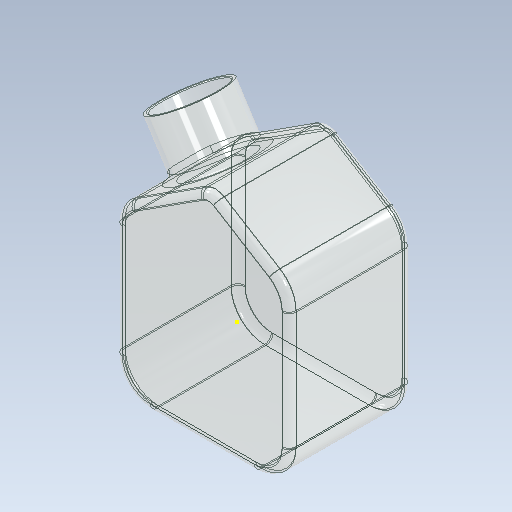
# Autodesk Inventor part: MediumBottle
Saved by Autodesk Inventor 2020 (Build 240168000, 168)
## iProperties
Created: 2023-04-07
Part Number: MediumBottle
Material: Glass
Document SubType Name: Modeling
Designer: DSOB
Density: 2.18 g/cm^3
Appearance: Clear
Author: DSOB
Autodesk Inventor part; units mm, degrees
ref_plane "XZ Plane" through (0, 0, 0) normal (0, 1, 0) x (-1, 0, 0)
ref_plane "XY Plane" through (0, 0, 0) normal (0, 0, 1) x (1, 0, 0)
sketch "Sketch1" plane through (0, 0, 0) normal (0, 0, 1) x (1, 0, 0)
  line L0 (0, 20) -> (0, 84.7083)
  line L1 (7.8208, 99.0171) -> (47.7041, 124.6026)
  line L2 (58.3547, 124.696) -> (90.5021, 104.8604)
  line L3 (100, 87.8397) -> (100, 20)
  line L4 (80, 0) -> (20, 0)
  arc A0 (0, 20) -> (20, 0) centre (20, 20) ccw
  arc A1 (80, 0) -> (100, 20) centre (80, 20) ccw
  arc A2 (100, 87.8397) -> (90.5021, 104.8604) centre (80, 87.8397) ccw
  arc A3 (7.8208, 99.0171) -> (0, 84.7083) centre (17, 84.7083) ccw
  arc A4 (58.3547, 124.696) -> (47.7041, 124.6026) centre (53.1036, 116.1857) ccw
  point P0 (0, 0)
  point P1 (0, 94)
  point P2 (53, 128)
  point P3 (100, 99)
  point P4 (100, 0)
  dimension "d0" = 100
  dimension "d1" = 128
  dimension "d2" = 99
  dimension "d3" = 94
  dimension "d4" = 53
  dimension "d5" = 20
  dimension "d6" = 20
  dimension "d7" = 20
  dimension "d8" = 17
  dimension "d9" = 10
  constraints: 10 end point, 10 point on circle, 10 point on line, 10 tangent, 5 centre point, 1 parallel, 1 perpendicular, 1 vertical
  measures "d0" distance between parallel lines of L3 L0
  measures "d1" distance from line of L4 point (53, 128)
  measures "d2" distance of point (100, 99) point (100, 0)
  measures "d3" distance of point (0, 0) point (0, 94)
  measures "d4" distance from line of point (53, 128) L0
  measures "d5" radius of A0
  measures "d6" radius of A1
  measures "d7" radius of A2
  measures "d8" radius of A3
  measures "d9" radius of A4
sketch "Sketch2" plane through (0, 0, 0) normal (1, 0, 0) x (0, 1, 0)
  point P0 (0, 0)
ref_plane "Work Plane1" through (53.975, 0, 0) normal (1, 0, 0) x (0, 1, 0)
sketch "Sketch3" plane through (53.975, 0, 0) normal (1, 0, 0) x (0, 1, 0)
  line L0 (0.8, 0) -> (0, 0)
  line L1 (0, 0) -> (0, 69)
  line L2 (0, 69) -> (0.8, 69)
  line L3 (0.8, 69) -> (0.8, 0)
  point P0 (0, 0)
  dimension "d11" = 69
  dimension "d12" = 0.8
  dimension "d13" = 0
  constraints: 8 end point, 2 parallel, 1 horizontal, 1 perpendicular
  measures "d11" distance of L2.end L0.start
  measures "d12" distance of L1.end L2.end
  measures "d13" distance from line of point (0, 0) L1
sweep "Sweep1" add profiles "Sketch3" path "Sketch1" path curves A4 L1 A3 L0 A0 L4 A1 L3 A2 L2
sketch "Sketch4" plane through (20, 0, 69) normal (0, 0, 1) x (1, 0, 0)
  line L0 (28.136, 123.9293) -> (-11.7473, 98.3437) projected
  arc A0 (37.9346, 124.0152) -> (28.136, 123.9293) centre (33.1036, 116.1857) ccw projected
  line L1 (70.0821, 104.1795) -> (37.9346, 124.0152) projected
  arc A1 (79.2, 87.8397) -> (70.0821, 104.1795) centre (60, 87.8397) ccw projected
  line L2 (79.2, 20) -> (79.2, 87.8397) projected
  arc A2 (60, 0.8) -> (79.2, 20) centre (60, 20) ccw projected
  line L3 (0, 0.8) -> (60, 0.8) projected
  arc A3 (-19.2, 20) -> (0, 0.8) centre (0, 20) ccw projected
  line L4 (-19.2, 84.7083) -> (-19.2, 20) projected
  arc A4 (-11.7473, 98.3437) -> (-19.2, 84.7083) centre (-3, 84.7083) ccw projected
  arc A5 (-12.1792, 99.0171) -> (-20, 84.7083) centre (-3, 84.7083) ccw projected
  line L5 (-20, 84.7083) -> (-20, 20) projected
  arc A6 (-20, 20) -> (0, 0) centre (0, 20) ccw projected
  line L6 (0, 0) -> (60, 0) projected
  arc A7 (60, 0) -> (80, 20) centre (60, 20) ccw projected
  line L7 (80, 20) -> (80, 87.8397) projected
  arc A8 (80, 87.8397) -> (70.5021, 104.8604) centre (60, 87.8397) ccw projected
  line L8 (70.5021, 104.8604) -> (38.3547, 124.696) projected
  arc A9 (38.3547, 124.696) -> (27.7041, 124.6026) centre (33.1036, 116.1857) ccw projected
  line L9 (27.7041, 124.6026) -> (-12.1792, 99.0171) projected
  point P0 (-20, 0)
extrude "Extrusion1" add sketch "Sketch4" along normal blind 0.8 contours A0 L1 A1 L2 A2 L3 A3 L4 A4 L0 | L9 A9 L8 A8 L7 A7 L6 A6 L5 A5
fillet "Fillet2" radius 4 10 edges at (53.0229, 125.3853, 69) (28.1944, 111.1365, 69) (2.7848, 92.4779, 69) (0.8, 52.3541, 69) (6.4235, 6.4235, 69) (50, 0.8, 69) (93.5765, 6.4235, 69) (99.2, 53.9198, 69) (96.7663, 97.1955, 69) (74.0083, 114.0974, 69)
fillet "Fillet3" radius 4 10 edges at (2.0828, 92.8616, 69.8) (0, 52.3541, 69.8) (5.8579, 5.8579, 69.8) (50, 0, 69.8) (94.1421, 5.8579, 69.8) (100, 53.9198, 69.8) (97.4649, 97.5854, 69.8) (74.4284, 114.7782, 69.8) (53.0159, 126.1853, 69.8) (27.7624, 111.8099, 69.8)
sketch "Sketch5" plane through (80, 0, 0) normal (0, 0, -1) x (-1, 0, 0)
  line L0 (32.2959, 124.6026) -> (72.1792, 99.0171) projected
  arc A0 (32.2959, 124.6026) -> (21.6453, 124.696) centre (26.8964, 116.1857) ccw projected
  line L1 (-10.5021, 104.8604) -> (21.6453, 124.696) projected
  arc A1 (-10.5021, 104.8604) -> (-20, 87.8397) centre (0, 87.8397) ccw projected
  line L2 (-20, 20) -> (-20, 87.8397) projected
  arc A2 (-20, 20) -> (0, 0) centre (0, 20) ccw projected
  line L3 (60, 0) -> (0, 0) projected
  arc A3 (60, 0) -> (80, 20) centre (60, 20) ccw projected
  line L4 (80, 84.7083) -> (80, 20) projected
  arc A4 (80, 84.7083) -> (72.1792, 99.0171) centre (63, 84.7083) ccw projected
  arc A5 (79.2, 84.7083) -> (71.7473, 98.3437) centre (63, 84.7083) ccw projected
  line L5 (79.2, 84.7083) -> (79.2, 20) projected
  arc A6 (60, 0.8) -> (79.2, 20) centre (60, 20) ccw projected
  line L6 (60, 0.8) -> (0, 0.8) projected
  arc A7 (-19.2, 20) -> (0, 0.8) centre (0, 20) ccw projected
  line L7 (-19.2, 20) -> (-19.2, 87.8397) projected
  arc A8 (-10.0821, 104.1795) -> (-19.2, 87.8397) centre (0, 87.8397) ccw projected
  line L8 (-10.0821, 104.1795) -> (22.0654, 124.0152) projected
  arc A9 (31.864, 123.9293) -> (22.0654, 124.0152) centre (26.8964, 116.1857) ccw projected
  line L9 (31.864, 123.9293) -> (71.7473, 98.3437) projected
  point P0 (80, 0)
extrude "Extrusion2" add sketch "Sketch5" along normal blind 0.8 contours L0 A4 L4 A3 L3 A2 L2 A1 L1 A0 | L5 A6 L6 A7 L7 A8 L8 A9 L9 A5
ref_plane "Work Plane3" through (20, 0, 41.225) normal (0, 0, 1) x (1, 0, 0)
fillet "Fillet4" radius 4 10 edges at (53.0229, 125.3853, 0) (28.1944, 111.1365, 0) (2.7848, 92.4779, 0) (0.8, 52.3541, 0) (6.4235, 6.4235, 0) (50, 0.8, 0) (93.5765, 6.4235, 0) (99.2, 53.9198, 0) (96.7663, 97.1955, 0) (74.0083, 114.0974, 0)
fillet "Fillet5" radius 4 10 edges at (94.1421, 5.8579, -0.8) (50, 0, -0.8) (5.8579, 5.8579, -0.8) (0, 52.3541, -0.8) (2.0828, 92.8616, -0.8) (27.7624, 111.8099, -0.8) (53.0159, 126.1853, -0.8) (74.4284, 114.7782, -0.8) (97.4649, 97.5854, -0.8) (100, 53.9198, -0.8)
sketch "Sketch6" plane through (7.8208, 99.0171, 65.8) normal (-0.5399547, 0.8416941, 0) x (0.8416941, 0.5399547, 0)
  circle A0 centre (20, 30.1664) radius 18.5
  line L0 (0, 62.6) -> (0, 0) projected
  line L1 (47.3846, 61.8) -> (47.3846, 0.8) projected
  circle A1 centre (20, 30.1664) radius 20.5
  point P0 (-60.0474, 65.8)
  point P1 (0, 34.6664)
  point P2 (0, 25.6664)
  dimension "d26" = 20
  dimension "d27" = 37
  dimension "d28" = 41
  constraints: 2 centre point, 1 coincident
  measures "d26" distance from line of L0 A0.centre
  measures "d27" diameter of A0
  measures "d28" diameter of A1
extrude "Extrusion3" add sketch "Sketch6" along normal blind 30 and the other way blind 0.8
fillet "Fillet6" radius 4 1 edges at (41.9094, 120.8853, 35.6336)
chamfer "Chamfer1" distance 0.5 angle 45 1 edges at (-7.1153, 125.0779, 35.6336)
sketch "Sketch7" plane through (24.6547, 109.8162, 35.6336) normal (-0.5399547, 0.8416941, 0) x (0.8416941, 0.5399547, 0)
  circle A0 centre (0, 0) radius 18.5 projected
  point P0 (-80.0474, 35.6336)
extrude "Extrusion4" cut sketch "Sketch7" against normal up to next
body "Solid1"
